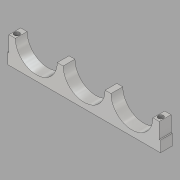
# Autodesk Inventor part: Tube Holder Halve
Saved by Autodesk Inventor 2017 (Build 210142000, 142)
## iProperties
Created: 2016-12-06
Part Number: Tube Holder Halve
Material: Aluminum 6061-AHC
Document SubType Name: Modeling
Designer: qupec
Density: 2.7 g/cm^3
Appearance: Aluminum - Dark
Mass: 20.4912 g
Surface Area: 43.8677 cm^2
Volume: 7.58934 cm^3
Author: qupec
Autodesk Inventor part; units mm, degrees
ref_plane "YZ Plane" through (0, 0, 0) normal (1, 0, 0) x (0, 1, 0)
ref_plane "XZ Plane" through (0, 0, 0) normal (0, 1, 0) x (-1, 0, 0)
ref_plane "XY Plane" through (0, 0, 0) normal (0, 0, 1) x (1, 0, 0)
sketch "Sketch1" plane through (0, 0, 0) normal (0, 0, 1) x (1, 0, 0)
  line L0 (-41.148, 14.2875) -> (41.148, 14.2875)
  line L1 (41.148, 14.2875) -> (41.148, -14.2875)
  line L2 (41.148, -14.2875) -> (-41.148, -14.2875)
  line L3 (-41.148, -14.2875) -> (-41.148, 14.2875)
  point P0 (0, 0)
  dimension "d0" = 82.296
  dimension "d1" = 41.148
  dimension "d2" = 14.2875
  dimension "d3" = 28.575
  constraints: 8 end point, 2 parallel, 1 horizontal, 1 perpendicular
  measures "d0" distance of L0.start L0.end
  measures "d1" distance from line of point (0, 0) L3
  measures "d2" distance from line of point (0, 0) L2
  measures "d3" distance of L2.end L0.start
extrude "Extrusion1" add sketch "Sketch1" along normal mid plane 6.35
sketch "Sketch2" plane through (0, 0, 3.175) normal (0, 0, 1) x (1, 0, 0)
  circle A0 centre (-25.781, 0) radius 11.303
  circle A1 centre (0, 0) radius 11.303
  line L0 (41.148, -14.2875) -> (41.148, 14.2875) projected
  circle A2 centre (25.781, 0) radius 11.303
  line L1 (-41.148, 14.2875) -> (-41.148, -14.2875) projected
  line L2 (-41.148, 0) -> (41.148, 0) construction
  line L3 (41.148, 14.2875) -> (-41.148, 14.2875) projected
  point P0 (0, 0)
  dimension "d6" = 22.606
  dimension "d9" = 22.606
  dimension "d11" = 22.606
  dimension "d14" = 25.781
  dimension "d21" = 82.296
  dimension "d22" = 25.781
  dimension "d45" = 0
  dimension "d84" = 3.175
  constraints: 3 centre point, 3 midpoint, 2 end point, 1 point on line
  measures "d6" diameter of A0
  measures "d9" diameter of A1
  measures "d11" diameter of A2
  measures "d14" distance of A1.centre A0.centre
  measures "d21" distance of L0.end L1.start
  measures "d22" distance of A2.centre A1.centre
  measures "d45" distance of point (0, 0) A1.centre
sketch "Sketch4" plane through (-41.148, -14.2875, -3.175) normal (-1, 0, 0) x (0, 0, 1)
  line L0 (0, 0) -> (0, 28.575) projected
  line L1 (6.35, 28.575) -> (6.35, 0) projected
  line L2 (0, 22.6695) -> (6.35, 22.6695)
  line L3 (6.35, 22.6695) -> (6.35, 5.9055)
  line L4 (6.35, 5.9055) -> (0, 5.9055)
  line L5 (0, 5.9055) -> (0, 22.6695)
  line L6 (6.35, 0) -> (0, 0) projected
  line L7 (0, 28.575) -> (6.35, 28.575) projected
  point P0 (3.175, 14.2875)
  dimension "d30" = 8.382
  dimension "d31" = 16.764
  dimension "d79" = 28.575
  constraints: 8 end point, 2 parallel, 1 horizontal, 1 perpendicular, 1 point on line, 2 other
  measures "d30" distance from line of point (3.175, 14.287) L4
  measures "d31" distance between parallel lines of L4 L2
  measures "d79" distance between parallel lines of L6 L7
extrude "Extrusion3" cut sketch "Sketch4" against normal blind 0.635 contours L0 L2 L1 L4
mirror "Mirror1" about plane through (0, 0, 0) normal (1, 0, 0) of "Extrusion3"
sketch "Sketch5" plane through (0, 0, 3.175) normal (0, 0, 1) x (1, 0, 0)
  circle A0 centre (0, 9.7155) radius 3.175 construction
  line L0 (41.148, 14.2875) -> (-41.148, 14.2875) projected
  line L1 (-21.5766, 0) -> (40.513, 0) construction
  line L2 (40.513, 8.382) -> (40.513, -8.382) projected
  circle A1 centre (0, -9.7155) radius 3.175 construction
  circle A2 centre (-36.576, 9.7155) radius 3.175
  circle A3 centre (36.576, -9.7155) radius 3.175
  line L3 (-41.148, 14.2875) -> (-41.148, 8.382) projected
  line L4 (41.148, -8.382) -> (41.148, -14.2875) projected
  line L5 (41.148, -14.2875) -> (-41.148, -14.2875) projected
  point P0 (0, 0)
  point P1 (40.513, -8.382)
  point P2 (43.815, 14.2875)
  point P3 (43.815, -14.2875)
  dimension "d34" = 6.35
  dimension "d35" = 4.572
  dimension "d48" = 6.35
  dimension "d49" = 6.35
  dimension "d50" = 4.572
  dimension "d51" = 4.572
  dimension "d52" = 4.572
  dimension "d53" = 4.572
  constraints: 4 centre point, 2 end point, 1 symmetric about line, 3 other
  measures "d34" diameter of A0
  measures "d35" distance from line of L0 A0.centre
  measures "d48" diameter of A2
  measures "d49" diameter of A3
  measures "d50" distance from line of L0 A2.centre
  measures "d51" distance from line of L3 A2.centre
  measures "d52" distance from line of L4 A3.centre
  measures "d53" distance from line of L5 A3.centre
extrude "Extrusion4" [suppressed]
sketch "Sketch7" plane through (-41.148, -14.2875, 3.175) normal (0, -1, 0) x (1, 0, 0)
  line L0 (27.178, -14.605) -> (55.118, -14.605)
  line L1 (55.118, -14.605) -> (55.118, 8.255)
  line L2 (55.118, 8.255) -> (27.178, 8.255)
  line L3 (27.178, 8.255) -> (27.178, -14.605)
  point P0 (41.148, -3.175)
  dimension "d39" = 27.94
  dimension "d40" = 22.86
  dimension "d41" = 11.43
  dimension "d42" = 13.97
  constraints: 8 end point, 2 parallel, 1 horizontal, 1 perpendicular
  measures "d39" distance of L0.start L0.end
  measures "d40" distance of L2.end L0.start
  measures "d41" distance from line of point (41.148, -3.175) L0
  measures "d42" distance from line of point (41.148, -3.175) L1
extrude "Extrusion5" [suppressed]
sketch "Sketch10" plane through (0, 0, -3.175) normal (0, 0, -1) x (-1, 0, 0)
  circle A0 centre (36.576, -9.7155) radius 3.175
  line L0 (-41.148, -14.2875) -> (41.148, -14.2875) projected
  line L1 (-41.148, -8.382) -> (-41.148, -14.2875) projected
  line L2 (40.513, -8.382) -> (40.513, 8.382) projected
  line L3 (41.148, -14.2875) -> (41.148, -8.382) projected
  point P0 (0, 0)
  point P1 (43.815, -14.2875)
  point P2 (43.815, 14.2875)
  point P3 (40.513, 8.382)
  dimension "d71" = 6.35
  dimension "d72" = 4.572
  dimension "d81" = 4.572
  constraints: 1 centre point, 1 other
  measures "d71" diameter of A0
  measures "d72" distance from line of L0 A0.centre
  measures "d81" distance from line of L3 A0.centre
extrude "Extrusion9" cut sketch "Sketch10" against normal blind 1.27
extrude "Extrusion6" cut sketch "Sketch2" against normal blind 25.4
sketch "Sketch8" plane through (0, 0, -3.175) normal (0, 0, -1) x (-1, 0, 0)
  line L0 (40.513, 8.382) -> (40.513, -8.382) construction
  line L1 (40.513, 0) -> (-40.513, 0)
  line L2 (-40.513, 8.382) -> (-40.513, -8.382) construction
  line L3 (41.148, 14.2875) -> (-41.148, 14.2875) projected
  line L4 (41.148, 8.382) -> (41.148, 14.2875) projected
  line L5 (-41.148, 14.2875) -> (-41.148, 8.382) projected
  line L6 (-40.513, 8.382) -> (-40.513, 0)
  line L7 (-41.148, 8.382) -> (-40.513, 8.382) projected
  line L8 (40.513, 8.382) -> (40.513, 0)
  line L9 (40.513, 8.382) -> (41.148, 8.382) projected
  point P0 (0, 0)
  point P1 (40.513, -8.382)
  point P2 (-40.513, -8.382)
  point P3 (43.815, 14.2875)
  point P4 (43.815, -14.2875)
  point P5 (-43.815, 14.2875)
  point P6 (-43.815, -14.2875)
  constraints: 6 end point, 2 vertical, 4 other
extrude "Extrusion7" cut sketch "Sketch8" against normal through all
sketch "Sketch9" plane through (-41.148, -14.2875, 3.175) normal (0, -1, 0) x (1, 0, 0)
  circle A0 centre (2.3495, -2.54) radius 1.4224
  line L0 (0, 0) -> (0, -6.35) projected
  line L1 (4.064, 0) -> (26.67, 0) projected
  line L2 (0.635, 0) -> (0.635, -6.35) projected
  line L3 (7.747, -5.08) -> (1.397, -5.08) projected
  line L4 (7.747, -6.35) -> (1.397, -6.35) projected
  point P0 (41.148, -3.175)
  dimension "d56" = 2.8448
  dimension "d58" = 3.429
  dimension "d60" = 1.7145
  dimension "d74" = 5.08
  dimension "d75" = 2.54
  constraints: 1 centre point
  measures "d56" diameter of A0
  measures "d58" distance from line of L1.start L2
  measures "d60" horizontal distance of L1.start A0.centre
  measures "d74" distance between parallel lines of L3 L1
  measures "d75" distance from line of L1 A0.centre
extrude "Extrusion8" cut sketch "Sketch9" against normal through all
mirror "Mirror2" about plane through (0, 0, 0) normal (1, 0, 0) of "Extrusion8"
thread "Thread1" size "5-40 UNC" class "2B" standard "ANSI Unified Screw Threads" length 25.4 offset 6.35
thread "Thread2" size "5-40 UNC" class "2B" standard "ANSI Unified Screw Threads" length 25.4 offset 6.35
sketch "Sketch11" plane through (0, 0, 3.175) normal (0, 0, 1) x (1, 0, 0)
  circle A0 centre (-36.576, -9.7155) radius 3.175 projected
  circle A1 centre (-36.576, -9.7155) radius 1.4224
  point P0 (0, 0)
  dimension "d82" = 2.8448
  constraints: 1 centre point, 1 coincident
  measures "d82" diameter of A1
equation "\"d1\" = 0.5 * d0"
equation "\"d2\" = 0.5 * d3"
equation "\"d9\" = d7"
equation "\"d11\" = d9"
equation "\"d22\" = d14"
equation "\"d30\" = 0.5 * d31"
equation "\"d41\" = 0.5 * d40"
equation "\"d42\" = 0.5 * d39"
equation "\"d60\" = 0.5 * d58"
equation "\"d75\" = 0.5 * d74"
equation "\"d7\" = d6"
body "Solid1"
